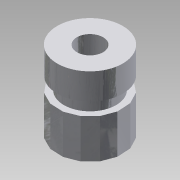
# Autodesk Inventor part: servo 2
Saved by Autodesk Inventor 2016 (Build 200138000, 138)
## iProperties
Created: 2016-07-30
Part Number: servo 2
Material: Generic
Document SubType Name: Modeling
Designer: julianesteban
Density: 1 g/cm^3
Appearance: Default
Author: julianesteban
Autodesk Inventor part; units mm, degrees
ref_plane "YZ Plane" through (0, 0, 0) normal (1, 0, 0) x (0, 1, 0)
ref_plane "XZ Plane" through (0, 0, 0) normal (0, 1, 0) x (-1, 0, 0)
ref_plane "XY Plane" through (0, 0, 0) normal (0, 0, 1) x (1, 0, 0)
sketch "Sketch1" plane through (0, 0, 0) normal (0, 0, 1) x (1, 0, 0)
  line L0 (2.4094, 0.6671) -> (2.4724, -0.3706)
  line L1 (2.4724, -0.3706) -> (2.1079, -1.3442)
  line L2 (2.1079, -1.3442) -> (1.3789, -2.0853)
  line L3 (1.3789, -2.0853) -> (0.4116, -2.4659)
  line L4 (0.4116, -2.4659) -> (-0.627, -2.4201)
  line L5 (-0.627, -2.4201) -> (-1.5571, -1.9558)
  line L6 (-1.5571, -1.9558) -> (-2.218, -1.1534)
  line L7 (-2.218, -1.1534) -> (-2.4954, -0.1515)
  line L8 (-2.4954, -0.1515) -> (-2.3413, 0.8765)
  line L9 (-2.3413, 0.8765) -> (-1.7824, 1.753)
  line L10 (-1.7824, 1.753) -> (-0.9153, 2.3264)
  line L11 (-0.9153, 2.3264) -> (0.1101, 2.4976)
  line L12 (0.1101, 2.4976) -> (1.1165, 2.2369)
  line L13 (1.1165, 2.2369) -> (1.9297, 1.5894)
  line L14 (1.9297, 1.5894) -> (2.4094, 0.6671)
  circle A0 centre (0, 0) radius 1
  dimension "d1" = 2
  constraints: 30 end point, 1 centre point, 1 coincident, 31 other
  measures "d1" diameter of A0
extrude "Extrusion1" add sketch "Sketch1" along normal blind 3
sketch "Sketch2" plane through (0, 0, 3) normal (0, 0, 1) x (1, 0, 0)
  circle A0 centre (0, 0) radius 1 projected
  line L0 (2.4724, -0.3706) -> (2.4094, 0.6671) projected
  line L1 (2.4094, 0.6671) -> (1.9297, 1.5894) projected
  line L2 (1.9297, 1.5894) -> (1.1165, 2.2369) projected
  line L3 (1.1165, 2.2369) -> (0.1101, 2.4976) projected
  line L4 (0.1101, 2.4976) -> (-0.9153, 2.3264) projected
  line L5 (-0.9153, 2.3264) -> (-1.7824, 1.753) projected
  line L6 (-1.7824, 1.753) -> (-2.3413, 0.8765) projected
  line L7 (-2.3413, 0.8765) -> (-2.4954, -0.1515) projected
  line L8 (-2.4954, -0.1515) -> (-2.218, -1.1534) projected
  line L9 (-2.218, -1.1534) -> (-1.5571, -1.9558) projected
  line L10 (-1.5571, -1.9558) -> (-0.627, -2.4201) projected
  line L11 (-0.627, -2.4201) -> (0.4116, -2.4659) projected
  line L12 (0.4116, -2.4659) -> (1.3789, -2.0853) projected
  line L13 (1.3789, -2.0853) -> (2.1079, -1.3442) projected
  line L14 (2.1079, -1.3442) -> (2.4724, -0.3706) projected
  circle A1 centre (0, 0) radius 2
  dimension "d4" = 4
  constraints: 1 centre point, 1 coincident
  measures "d4" diameter of A1
extrude "Extrusion2" add sketch "Sketch2" along normal blind 1 contours A1
sketch "Sketch3" plane through (0, 0, 4) normal (0, 0, 1) x (1, 0, 0)
  circle A0 centre (0, 0) radius 1 projected
  circle A1 centre (0, 0) radius 2 projected
  circle A2 centre (0, 0) radius 2.5
  dimension "d7" = 5
  constraints: 1 centre point, 1 coincident
  measures "d7" diameter of A2
extrude "Extrusion3" add sketch "Sketch3" along normal blind 2 contours A1 | A2
body "Solid1"
